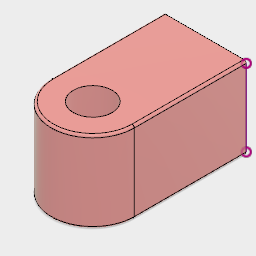
BabyCrib_RailGuide (Autodesk Fusion 360 design; units mm, degrees)
Autodesk Fusion 360 part; units mm, degrees
sketch "Sketch1" plane through (0, 0, 0) normal (0, 1, 0) x (1, 0, 0)
  line L0 (0, 0) -> (18.4, 0)
  line L1 (18.4, 0) -> (18.4, -34)
  line L2 (18.4, -34) -> (0, -34)
  line L3 (0, -34) -> (0, 0)
  circle A0 centre (9.2, -24.8) radius 9.2
  circle A1 centre (9.2, -24.8) radius 4.3
  dimension "d1" = 18.4
  dimension "d2" = 34
  dimension "d3" = 4.9
  measures "d1" distance of L0.start L0.end
  measures "d2" distance of L0.start L2.end
extrude "Extrude2" add sketch "Sketch1" along normal blind 18 contours L0 L1 L3 A0 | A0
fillet "Fillet1" radius 0.5 6 edges at (18.4, 0, 12.4) (9.2, 0, 34) (0, 0, 12.4) (0, 18, 12.4) (9.2, 18, 34) (18.4, 18, 12.4)
sketch "Sketch2" plane through (0, 0, 0) normal (0, 0, 1) x (1, 0, 0)
  line L0 (18.4, 0.5) -> (18.4, 17.5)
sketch "Sketch3" plane through (0, 0, 0) normal (0, 0, 1) x (1, 0, 0)
  circle A0 centre (9.2, 9.2591) radius 2.3
  dimension "d9" = 4.6
  measures "d9" diameter of A0
extrude "Extrude3" cut sketch "Sketch3" along normal blind 17
